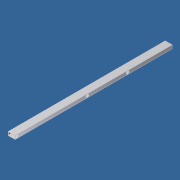
# Autodesk Inventor part: GE-12027-01
Saved by Autodesk Inventor 2012 (Build 160160000, 160)
## iProperties
Created: 2011-07-18
Part Number: GE-12027-01
Document SubType Name: Modeling
Designer: dfoster
Density: 1 g/cm^3
Description: Main Support
Material: Default
Title: Main Support
Author: dfoster
Autodesk Inventor part; units mm, degrees
ref_plane "YZ Plane" through (0, 0, 0) normal (1, 0, 0) x (0, 1, 0)
ref_plane "XZ Plane" through (0, 0, 0) normal (0, 1, 0) x (-1, 0, 0)
ref_plane "XY Plane" through (0, 0, 0) normal (0, 0, 1) x (1, 0, 0)
sketch "Sketch1" plane through (0, 0, 0) normal (0, 0, 1) x (1, 0, 0)
  line L0 (0, 0) -> (88.9, 0)
  line L1 (88.9, 0) -> (88.9, 44.45)
  line L2 (88.9, 44.45) -> (0, 44.45)
  line L3 (0, 44.45) -> (0, 0)
  line L4 (3.175, 41.275) -> (85.725, 41.275)
  line L5 (85.725, 41.275) -> (85.725, 3.175)
  line L6 (85.725, 3.175) -> (3.175, 3.175)
  line L7 (3.175, 3.175) -> (3.175, 41.275)
  dimension "d0" = 3.175
  dimension "d1" = 88.9
  dimension "d2" = 44.45
  constraints: 16 end point, 4 parallel, 2 perpendicular, 1 horizontal, 3 other
  measures "d0" distance between parallel lines of L4 L2
  measures "d1" distance of L1.end L2.end
  measures "d2" distance of L2.end L0.start
extrude "Extrusion1" add sketch "Sketch1" along normal blind 1981.2
hole "Hole1" at (88.9, 22.225, 1958.975) direction (-1, 0, 0) diameter 38.1 end through all
pattern_linear "Rectangular Pattern1" count 2 spacing 889 along (0, 0, -1) of "Hole1"
hole "Hole2" at (88.9, 22.225, 561.975) direction (-1, 0, 0) diameter 38.1 end through all
body "Solid1"
